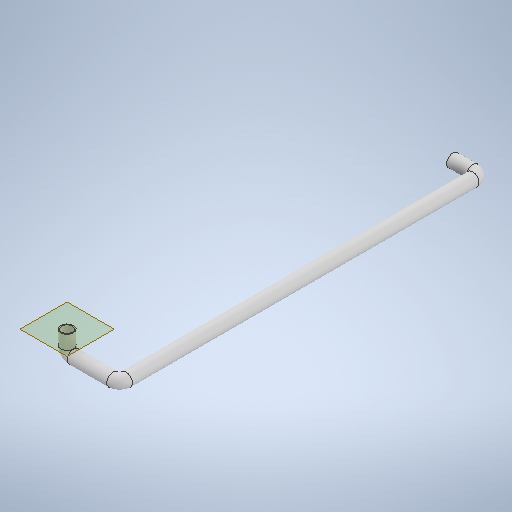
# Autodesk Inventor part: Pipe
Saved by Autodesk Inventor 2025.2 (Build 292293000, 293)
## iProperties
Created: 2025-05-29
Part Number: Pipe
Material: Generic
Document SubType Name: Modeling
Designer: Simon
Density: 1 g/cm^3
Appearance: Default
Author: Simon
Autodesk Inventor part; units mm, degrees
ref_plane "YZ Plane" through (0, 0, 0) normal (1, 0, 0) x (0, 1, 0)
ref_plane "XZ Plane" through (0, 0, 0) normal (0, 1, 0) x (-1, 0, 0)
ref_plane "XY Plane" through (0, 0, 0) normal (0, 0, 1) x (1, 0, 0)
ref_plane "Work Plane1" through (0, 0, 0) normal (0, -1, 0) x (1, 0, 0)
sketch "Sketch1" plane through (0, 0, 0) normal (0, -1, 0) x (1, 0, 0)
  circle A0 centre (0, 0) radius 3
  circle A1 centre (0, 0) radius 2.5
  dimension "d8" = 6
  dimension "d9" = 5
  constraints: 2 centre point, 2 coincident
  measures "d8" diameter of A0
  measures "d9" diameter of A1
sketch3d "3D Sketch1"
  line L0 (0, 0, 0) -> (0, -6.497, 0)
  arc A0 (0, -6.497, 0) -> (3, -9.497, 0) centre (3, -6.497, 0) ccw
  line L1 (3, -9.497, 0) -> (21.5, -9.497, 0)
  arc A1 (21.5, -9.497, 0) -> (24.5, -9.497, -3) centre (21.5, -9.497, -3) ccw
  line L2 (24.5, -9.497, -3) -> (24.5, -9.497, -164.75)
  arc A2 (24.5, -9.497, -164.75) -> (21.5, -9.497, -167.75) centre (21.5, -9.497, -164.75) ccw
  line L3 (21.5, -9.497, -167.75) -> (12.25, -9.497, -167.75)
  dimension "d0" = 6.497
  dimension "d1" = 3
  dimension "d2" = 90
  dimension "d3" = 18.5
  dimension "d4" = 90
  dimension "d5" = 161.75
  dimension "d6" = 90
  dimension "d7" = 9.25
sweep "Sweep1" add profiles "Sketch1" path "3D Sketch1"
body "Solid1"
